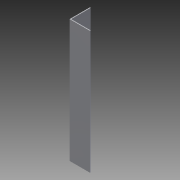
# Autodesk Inventor part: kątownik 1
Saved by Autodesk Inventor 2014 (Build 180170000, 170)
## iProperties
Created: 2013-08-20
Part Number: kątownik 1
Material: Aluminium 6061
Document SubType Name: Modeling
Designer: Kisieel
Density: 1 g/cm^3
Appearance: Aluminium — płaski
Author: Kisieel
Autodesk Inventor part; units mm, degrees
ref_plane "YZ Plane" through (0, 0, 0) normal (1, 0, 0) x (0, 1, 0)
ref_plane "XZ Plane" through (0, 0, 0) normal (0, 1, 0) x (-1, 0, 0)
ref_plane "XY Plane" through (0, 0, 0) normal (0, 0, 1) x (1, 0, 0)
sketch "Szkic1" plane through (0, 0, 0) normal (0, 0, 1) x (1, 0, 0)
  line L0 (-10.1243, 0) -> (60.0207, 0) projected
  line L1 (0, -10.1243) -> (0, 60.0207) projected
  line L2 (0, 50) -> (0, 0.5)
  line L3 (0.5, 0) -> (50, 0)
  line L4 (50, 2) -> (2.5, 2)
  line L5 (2, 2.5) -> (2, 50)
  line L6 (2, 50) -> (0, 50)
  line L7 (50, 0) -> (50, 2)
  arc A0 (2, 2.5) -> (2.5, 2) centre (2.5, 2.5) ccw
  arc A1 (0, 0.5) -> (0.5, 0) centre (0.5, 0.5) ccw
  point P0 (0, 0)
  dimension "d0" = 2
  dimension "d2" = 2
  dimension "d3" = 50
  dimension "d4" = 50
  dimension "d5" = 0.5
  constraints: 12 end point, 4 point on circle, 4 point on line, 4 tangent, 2 centre point, 2 parallel, 2 perpendicular, 1 collinear, 1 equal radius
  measures "d0" distance between parallel lines of L5 L2
  measures "d2" distance between parallel lines of L0 L4
  measures "d3" distance between parallel lines of L1 L7
  measures "d4" distance between parallel lines of L0 L6
  measures "d5" radius of A0
extrude "Wyciągnięcie proste1" add sketch "Szkic1" along normal blind 300 contours A1 L1 L6 L5 A0 L4 L7 L0
